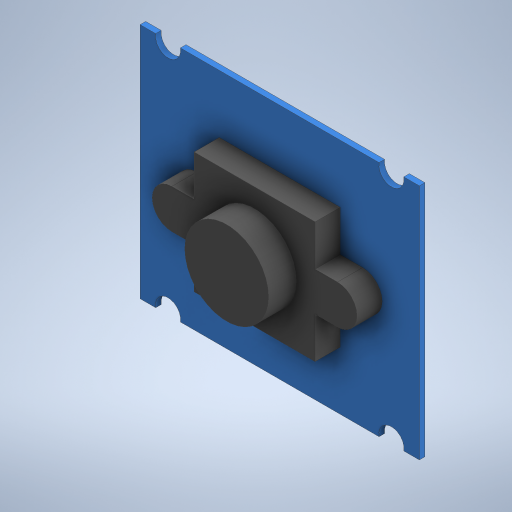
# Autodesk Inventor part: 카메라
Saved by Autodesk Inventor 2023 (Build 270158000, 158)
## iProperties
Created: 2022-11-10
Part Number: 카메라
Material: 일반
Document SubType Name: Modeling
Designer: user
Density: 1 g/cm^3
Appearance: 기본값
Author: user
Autodesk Inventor part; units mm, degrees
ref_plane "YZ Plane" through (0, 0, 0) normal (1, 0, 0) x (0, 1, 0)
ref_plane "XZ Plane" through (0, 0, 0) normal (0, 1, 0) x (-1, 0, 0)
ref_plane "XY Plane" through (0, 0, 0) normal (0, 0, 1) x (1, 0, 0)
sketch "스케치1" plane through (0, 0, 0) normal (0, 0, 1) x (1, 0, 0)
  line L0 (-15, 12.75) -> (15, 12.75)
  line L1 (15, 12.75) -> (15, -12.75)
  line L2 (15, -12.75) -> (-15, -12.75)
  line L3 (-15, -12.75) -> (-15, 12.75)
  line L4 (-15, 12.75) -> (15, -12.75) construction
  line L5 (15, 12.75) -> (-15, -12.75) construction
  point P0 (0, 0)
  dimension "d0" = 30
  dimension "d1" = 25.5
  constraints: 12 end point, 2 midpoint, 2 parallel, 1 horizontal, 1 perpendicular
  measures "d0" distance of L1.end L2.end
  measures "d1" distance of L0.end L1.end
extrude "돌출1" add sketch "스케치1" along normal blind 0.6
sketch "스케치2" plane through (0, 0, 0.6) normal (0, 0, 1) x (1, 0, 0)
  line L0 (-12, 12.5) -> (12, 12.5) construction
  line L1 (12, 12.5) -> (12, -12.5) construction
  line L2 (12, -12.5) -> (-12, -12.5) construction
  line L3 (-12, -12.5) -> (-12, 12.5) construction
  line L4 (-12, 12.5) -> (12, -12.5) construction
  line L5 (12, 12.5) -> (-12, -12.5) construction
  circle A0 centre (-12, 12.5) radius 1.35
  line L6 (0, 0) -> (2.9339, 0)
  line L7 (0, 0) -> (0, 3.0969)
  circle A1 centre (12, 12.5) radius 1.35
  circle A2 centre (-12, -12.5) radius 1.35
  circle A3 centre (12, -12.5) radius 1.35
  dimension "d4" = 24
  dimension "d5" = 25
  dimension "d6" = 2.7
  constraints: 16 end point, 4 centre point, 3 symmetric about line, 2 horizontal, 2 midpoint, 2 parallel, 1 coincident, 1 perpendicular, 1 vertical, 3 other
  measures "d4" distance of L1.end L2.end
  measures "d5" distance of L0.end L1.end
  measures "d6" diameter of A0
extrude "돌출2" cut sketch "스케치2" against normal blind 0.6
sketch "스케치3" plane through (0, 0, 0.6) normal (0, 0, 1) x (1, 0, 0)
  line L0 (-6.5, 6.5) -> (6.5, 6.5)
  line L1 (6.5, 6.5) -> (6.5, -6.5)
  line L2 (6.5, -6.5) -> (-6.5, -6.5)
  line L3 (-6.5, -6.5) -> (-6.5, 6.5)
  line L4 (-6.5, 6.5) -> (6.5, -6.5) construction
  line L5 (6.5, 6.5) -> (-6.5, -6.5) construction
  circle A0 centre (8.9, 0) radius 2.1
  line L6 (8.9, 2.1) -> (6.5, 2.1)
  line L7 (8.9, -2.1) -> (6.5, -2.1)
  line L8 (0, 0) -> (0, 1.8337)
  circle A1 centre (-8.9, 0) radius 2.1
  line L9 (-8.9, 2.1) -> (-6.5, 2.1)
  line L10 (-8.9, -2.1) -> (-6.5, -2.1)
  dimension "d9" = 13
  dimension "d10" = 13
  dimension "d11" = 4.2
  dimension "d12" = 17.8
  constraints: 22 end point, 5 symmetric about line, 4 point on circle, 3 perpendicular, 2 centre point, 2 midpoint, 2 parallel, 2 point on line, 2 tangent, 1 horizontal, 1 horizontal alignment, 1 vertical, 1 other
  measures "d9" distance of L1.end L2.end
  measures "d10" distance of L0.end L1.end
  measures "d11" diameter of A0
  measures "d12" distance of A0.centre A1.centre
extrude "돌출3" add sketch "스케치3" along normal blind 2.7
sketch "스케치4" plane through (0, 0, 3.3) normal (0, 0, 1) x (1, 0, 0)
  circle A0 centre (0, 0) radius 4.5
  dimension "d15" = 9
  constraints: 1 centre point, 1 coincident
  measures "d15" diameter of A0
extrude "돌출4" add sketch "스케치4" along normal blind 3
